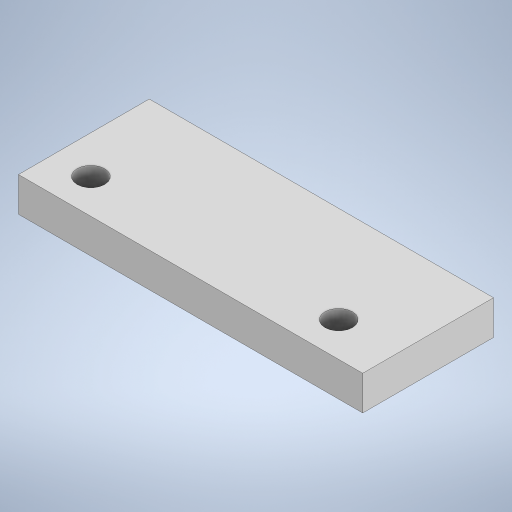
# Autodesk Inventor part: Fuhrungschiene
Saved by Autodesk Inventor 2023.2 (Build 272271000, 271)
## iProperties
Created: 2023-02-07
Part Number: Fuhrungschiene
Material: Generic
Document SubType Name: Modeling
Designer: Ayush
Density: 1 g/cm^3
Appearance: Default
Author: Ayush
Autodesk Inventor part; units mm, degrees
ref_plane "YZ Plane" through (0, 0, 0) normal (1, 0, 0) x (0, 1, 0)
ref_plane "XZ Plane" through (0, 0, 0) normal (0, 1, 0) x (-1, 0, 0)
ref_plane "XY Plane" through (0, 0, 0) normal (0, 0, 1) x (1, 0, 0)
sketch "Sketch1" plane through (0, 0, 0) normal (0, 1, 0) x (-1, 0, 0)
  line L0 (-25, 9.5) -> (25, 9.5)
  line L1 (25, 9.5) -> (25, -9.5)
  line L2 (25, -9.5) -> (-25, -9.5)
  line L3 (-25, -9.5) -> (-25, 9.5)
  line L4 (-25, 9.5) -> (25, -9.5) construction
  line L5 (25, 9.5) -> (-25, -9.5) construction
  circle A0 centre (19.484, 4.5) radius 2
  circle A1 centre (-16.516, 4.5) radius 2
  point P0 (0, 0)
  dimension "d0" = 50
  dimension "d1" = 19
  dimension "d2" = 4
  dimension "d3" = 4
  dimension "d4" = 36
  dimension "d5" = 5
  constraints: 12 end point, 2 centre point, 2 midpoint, 2 parallel, 1 horizontal, 1 horizontal alignment, 1 perpendicular
  measures "d0" distance of L1.end L2.end
  measures "d1" distance of L0.end L1.end
  measures "d2" diameter of A0
  measures "d3" diameter of A1
  measures "d4" distance of A1.centre A0.centre
  measures "d5" distance from line of L0 A0.centre
extrude "Extrusion1" add sketch "Sketch1" along normal blind 5
body "Solid1"
